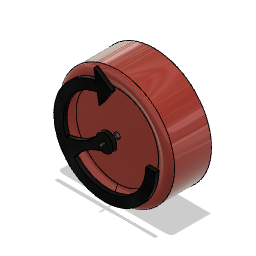
Micro stepper rotobrooch v5 (Autodesk Fusion 360 design; units mm, degrees)
Autodesk Fusion 360 part; units mm, degrees
ref_plane "WorkPlane1" through (0, 0, -96.52) normal (0, 0, 1) x (1, 0, 0)
mesh "Mesh1" [no effect]
ref_plane "WorkPlane1" through (0, 0, -9.6012) normal (0, 0, 1) x (1, 0, 0) in component "Backing"
sketch "Sketch1" plane through (0, 0, -9.6012) normal (0, 0, 1) x (1, 0, 0) in component "Backing"
  circle A0 centre (0.0091, 9.9958) radius 2.0003
  circle A1 centre (-0.0085, -0.0204) radius 15.3019
  dimension "d4" = 4.0005
  measures "d4" diameter of A0
extrude "Extrude1" add sketch "Sketch1" against normal blind 1.5875 makes body 1 in component "Backing"
sketch "Sketch2" plane through (0, 0, -9.6012) normal (0, 0, 1) x (1, 0, 0) in component "Backing"
  circle A0 centre (0.0091, 9.9958) radius 2.0003
  circle A1 centre (-0.0085, -0.0204) radius 15.3019
  point P0 (11.4411, 3.7804)
  point P1 (11.4411, -3.8606)
  point P2 (-11.4424, 3.7804)
  point P3 (-11.4424, -3.8606)
hole "Hole1" at (11.4411, 3.7804, -9.6012) at (-11.4424, 3.7804, -9.6012) at (-11.4424, -3.8606, -9.6012) at (11.4411, -3.8606, -9.6012) direction (0, 0, -1) diameter 1.5875 depth 1.5875 tip angle 180 bodies 1 in component "Backing"
sketch "Sketch3" plane through (0, 0, -9.6012) normal (0, 0, 1) x (1, 0, 0) in component "Backing"
  circle A0 centre (-11.4424, -3.8606) radius 0.7937
  circle A1 centre (11.4411, 3.7804) radius 0.7937
  circle A2 centre (-11.4424, 3.7804) radius 0.7937
  circle A3 centre (11.4411, -3.8606) radius 0.7937
  circle A4 centre (0.0091, 9.9958) radius 2.0003
  circle A5 centre (-0.0085, -0.0204) radius 15.3019
  point P0 (-13.4872, -0.0415)
  point P1 (13.5198, -0.0415)
hole "Hole2" at (-13.4872, -0.0415, -9.6012) at (13.5198, -0.0415, -9.6012) direction (0, 0, -1) diameter 2.5 depth 1.6002 tip angle 180 bodies 1 in component "Backing"
hole "Hole3" at (-8.9981, -8.9846, -9.6012) direction (0, 0, -1) diameter 3.175 depth 1.6002 tip angle 180 bodies 1 in component "Backing"
sketch "Sketch1 (2)" plane through (0, 0, 0) normal (0, 0, 1) x (1, 0, 0) in component "Housing"
  circle A0 centre (-0.0366, 5.9923) radius 22.225
  circle A1 centre (-0.0366, 5.9923) radius 1.1224
  dimension "d16" = 44.45
  constraint coincident A0.centre A1.centre
  measures "d16" diameter of A0
extrude "Extrude1'" add sketch "Sketch1 (2)" along normal blind 1.5875 separate body makes body 2 in component "Housing"
sketch "Sketch2 (2)" plane through (0, 0, 0) normal (0, 0, -1) x (-1, 0, 0) in component "Housing"
  circle A0 centre (0.0366, 5.9923) radius 1.1224
  circle A1 centre (0.0366, 5.9923) radius 22.225
  arc A2 (12.1918, -9.6929) -> (-12.2644, -9.5788) centre (0.0366, 5.9923) ccw
  arc A3 (-11.3853, -10.2347) -> (11.3066, -10.3405) centre (0.0085, -0.0204) ccw
  arc A4 (-12.2644, -9.5788) -> (12.1918, -9.6929) centre (0.0085, -0.0204) ccw
  dimension "d19" = 2.3813
  constraint concentric A0 A2
  constraint concentric A3 A4
  measures "d19" distance of A1 A2
extrude "Extrude2" add sketch "Sketch2 (2)" along normal up to surface (12.7762 mm away) contours A1 bodies 2 in component "Housing"
sketch "Sketch3 (2)" plane through (0, 0, 0) normal (1, 0, 0) x (0, 0, -1) in component "Housing"
  line L0 (-1.5875, 28.2173) -> (-1.5875, -16.2327)
  line L1 (-1.5875, 5.9923) -> (-11.8113, 5.9923) construction
  spline S0 degree 5 poles (-1.5875, -16.2327) (-1.6143, -16.2448) (-1.6696, -16.2609) (-1.7574, -16.2601) (-1.8843, -16.2091) (-2.0583, -16.0625) (-2.2432, -15.836) (-2.4301, -15.5373) (-2.6043, -15.18) (-2.7489, -14.7813) (-2.8475, -14.3592) (-2.8869, -13.931) (-2.8602, -13.5105) (-2.7706, -13.1062) (-2.6296, -12.721) (-2.4543, -12.3543) (-2.264, -12.003) (-2.0776, -11.6629) (-1.9109, -11.33) (-1.7735, -11.0018) (-1.6711, -10.6767) (-1.6189, -10.4184) (-1.5966, -10.2256) (-1.5893, -10.0974) (-1.5875, -10.0334) knots 0 0 0 0 0 0 0.05 0.1 0.15 0.2 0.25 0.3 0.35 0.4 0.45 0.5 0.55 0.6 0.65 0.7 0.75 0.8 0.85 0.9 0.95 1 1 1 1 1 1
  line L2 (-1.5875, -9.3997) -> (-1.5875, -16.2327)
  point P0 (-2.2003, -15.8774)
  point P1 (-2.8692, -13.8003)
  point P2 (-2.0947, -11.688)
  constraint midpoint L0 L1.start
  constraint perpendicular L0 L1
  constraint coincident L0 L2.start
  constraint parallel L0 L2
revolve "Revolve1" add sketch "Sketch3 (2)" angle 360 about axis through (0, 5.9923, 1.5875) along (0, 0, 1) bodies 2 in component "Housing"
sketch "Sketch2 (3)" plane through (0, 0, 0) normal (0, 0, 1) x (1, 0, 0) in component "Component"
  line L0 (16.0381, 5.9934) -> (19.6718, 5.9934)
  arc A0 (-3.4195, 25.3693) -> (19.6718, 5.9934) centre (-0.003, 5.9934) ccw
  line L1 (2.7319, 24.609) -> (-4.1129, 29.3021)
  line L2 (2.7319, 24.609) -> (-2.0545, 17.628)
  line L3 (-2.0545, 17.628) -> (-0.003, 5.9934) construction
  line L4 (-0.003, 5.9934) -> (-0.003, 18.9703) construction
  line L5 (-0.003, 18.9703) -> (-0.003, 15.9682) construction
  line L6 (-4.1129, 29.3021) -> (-3.4195, 25.3693)
  line L7 (-2.7885, 21.7907) -> (-2.0545, 17.628)
  line L8 (-3.4195, 25.3693) -> (-2.7885, 21.7907) construction
  line L9 (-3.104, 23.58) -> (2.7319, 24.609) construction
  line L10 (-0.003, 5.9934) -> (-15.6038, -3.3425) construction
  arc A1 (-14.7111, 0.6187) -> (-3.2899, 6.5752) centre (-17.3998, 19.7021) ccw
  arc A2 (-1.0438, 2.8218) -> (-11.6911, -4.428) centre (3.8556, -15.817) ccw
  arc A3 (-1.0438, 2.8218) -> (-3.2899, 6.5752) centre (-0.003, 5.9934) ccw
  arc A4 (-14.7111, 0.6187) -> (-15.1426, 0.6918) centre (-15.6038, -3.3425) ccw
  arc A5 (-11.8306, -4.8428) -> (-11.6911, -4.428) centre (-15.6038, -3.3425) ccw
  arc A6 (-2.7885, 21.7907) -> (-15.1426, 0.6918) centre (-0.003, 5.9934) ccw
  arc A7 (-11.8306, -4.8428) -> (16.0381, 5.9934) centre (-0.003, 5.9934) ccw
  circle A8 centre (-0.003, 5.9934) radius 0.381
  dimension "d26" = 10
  dimension "d27" = 0.762
  constraint concentric A0 A6
  constraint perpendicular L1 L2
  constraint coincident A0.centre L3.end
  constraint parallel L3 L6
  constraint vertical L4
  constraint coincident L4 L5.end
  constraint parallel L4 L5
  constraint collinear L6 L7
  constraint parallel L7 L8
  constraint midpoint L8 L9.start
  constraint perpendicular L8 L9
  constraint concentric A3 A6
  constraint coincident L10.end A4.centre
  constraint symmetric L10 A1.start A2.end
  constraint symmetric L10 A1.end A2.start
  constraint symmetric L10 A1 A2
  constraint concentric A4 A5
  constraint coincident A5.start A6
  constraint concentric A6 A7
  constraint concentric A3 A8
  measures "d26" angle of L3 L5
  measures "d27" diameter of A8
extrude "Extrude1''" add sketch "Sketch2 (3)" along normal blind 1.5 separate body makes body 3 in component "Component"
component "Backing" placed x (1, 0, 0) y (0, 1, 0) z (0, 0, 1) at (0, 0, 0)
component "Housing" placed x (1, 0, 0) y (0, 1, 0) z (0, 0, 1) at (0, 0, 0)
component "Component" placed x (1, 0, 0) y (0, 1, 0) z (0, 0, 1) at (0, 0, 0)
